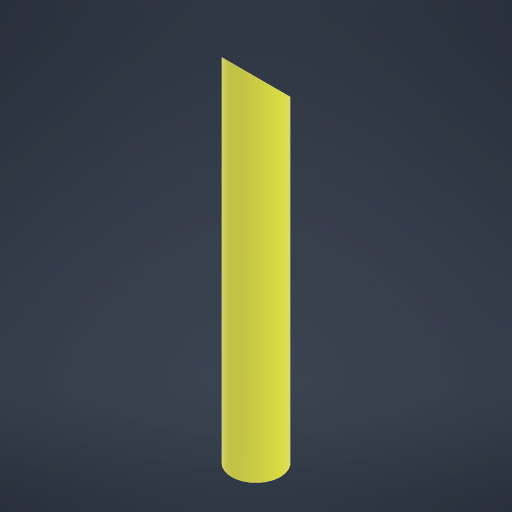
# Autodesk Inventor part: BUMP_Noodle1
Saved by Autodesk Inventor 2024.2 (Build 282272000, 272)
## iProperties
Created: 2024-08-07
Part Number: BUMP_Noodle1
Material: Pool Noodle
Document SubType Name: Modeling
Designer: Bryan
Density: 0.0830397 g/cm^3
Appearance: Yellow
Mass: 89.4245 g
Surface Area: 1194.81 cm^2
Volume: 1076.89 cm^3
Author: Bryan
Autodesk Inventor part; units mm, degrees
ref_plane "XZ Plane" through (0, 0, 0) normal (0, 1, 0) x (-1, 0, 0)
ref_plane "XY Plane" through (0, 0, 0) normal (0, 0, 1) x (1, 0, 0)
sketch "Sketch1" plane through (0, 0, 0) normal (0, 1, 0) x (-1, 0, 0)
  circle A0 centre (0, 0) radius 12.7
  circle A1 centre (0, 0) radius 31.75
  dimension "d0" = 63.5
  dimension "d1" = 25.4
  constraints: 2 centre point, 2 coincident
  measures "d0" diameter of A1
  measures "d1" diameter of A0
extrude "Extrusion1" add sketch "Sketch1" along normal blind 468.3125
ref_plane "Work Plane1" through (31.75, 0, 0) normal (1, 0, 0) x (0, 1, 0)
sketch "Sketch2" plane through (31.75, 0, 0) normal (1, 0, 0) x (0, 1, 0)
  line L0 (468.3125, -31.75) -> (468.3125, 31.75) projected
  line L1 (468.3125, 31.75) -> (404.8125, -31.75)
  line L2 (0, -31.75) -> (468.3125, -31.75) projected
  point P0 (0, 0)
  dimension "d4" = 45
  constraints: 2 end point, 1 point on line
  measures "d4" angle of L0 L1
extrude "Extrusion2" cut sketch "Sketch2" against normal blind 436.5625
body "Solid1"
